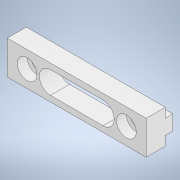
# Autodesk Inventor part: cameraModuleEnclosure
Saved by Autodesk Inventor 2022 (Build 260153000, 153)
## iProperties
Created: 2021-06-11
Part Number: cameraModuleEnclosure
Material: ABS Plastic
Document SubType Name: Modeling
Designer: tecware
Density: 1.06 g/cm^3
Appearance: Smooth - White
Mass: 91.0798 g
Surface Area: 506.315 cm^2
Volume: 85.9244 cm^3
Author: tecware
## iProperties of the stored document cameraModuleEnclosure_3DPrint.ipt
Created: 2021-06-17
Part Number: cameraModuleEnclosure_3DPrint
Material: Generic
Document SubType Name: Modeling
Designer: tecware
Density: 1 g/cm^3
Appearance: Default
Author: tecware
Autodesk Inventor part; units mm, degrees
ref_plane "YZ Plane" through (0, 0, 0) normal (1, 0, 0) x (0, 1, 0)
ref_plane "XZ Plane" through (0, 0, 0) normal (0, 1, 0) x (-1, 0, 0)
ref_plane "Work Plane15" through (0, 0, 83) normal (0, 0, 1) x (1, 0, 0)
sketch "Sketch35" plane through (0, 0, 83) normal (0, 0, 1) x (1, 0, 0)
  line L0 (-53.15, -19.2) -> (-22.85, -19.2)
  line L1 (-22.85, -19.2) -> (-22.85, -26.8)
  line L2 (-22.85, -26.8) -> (-53.15, -26.8)
  line L3 (-53.15, -26.8) -> (-53.15, -19.2)
  line L4 (-53.15, -26.8) -> (-22.85, -19.2) construction
  line L5 (-22.85, -26.8) -> (-53.15, -19.2) construction
  line L6 (-53.15, -23) -> (-49.35, -23) construction
  arc A0 (-49.35, -19.2) -> (-53.15, -23) centre (-49.35, -23) ccw
  arc A1 (-53.15, -23) -> (-49.35, -26.8) centre (-49.35, -23) ccw
  line L7 (-22.85, -23) -> (-26.65, -23) construction
  arc A2 (-22.85, -23) -> (-26.65, -19.2) centre (-26.65, -23) ccw
  arc A3 (-26.65, -26.8) -> (-22.85, -23) centre (-26.65, -23) ccw
  line L8 (-38, -26.8) -> (-38, -23)
  line L9 (-38, -26.8) -> (-34.2, -26.8) construction
  line L10 (-28, 6.8) -> (28, 6.8)
  line L11 (28, 6.8) -> (28, -6.8)
  line L12 (28, -6.8) -> (-28, -6.8)
  line L13 (-28, -6.8) -> (-28, 6.8)
  line L14 (-11.3, -22) -> (-6.85, -22) construction
  line L15 (3, -17.55) -> (3, -26.45)
  line L16 (-11.5, -17.5) -> (17.5, -17.5)
  line L17 (17.5, -17.5) -> (17.5, -26.5)
  line L18 (17.5, -26.5) -> (-11.5, -26.5)
  line L19 (-11.5, -26.5) -> (-11.5, -17.5)
  line L20 (-11.5, -22) -> (-7, -22)
  arc A4 (-7, -17.5) -> (-7, -26.5) centre (-7, -22) ccw
  arc A5 (13, -26.5) -> (13, -17.5) centre (13, -22) ccw
  line L21 (-15.1, 4.5) -> (15.1, 4.5)
  line L22 (15.1, 4.5) -> (15.1, -4.5)
  line L23 (15.1, -4.5) -> (-15.1, -4.5)
  line L24 (-15.1, -4.5) -> (-15.1, 4.5)
  line L25 (-15.1, 0) -> (-10.6, 0)
  arc A6 (-10.6, 4.5) -> (-10.6, -4.5) centre (-10.6, 0) ccw
  arc A7 (10.6, -4.5) -> (10.6, 4.5) centre (10.6, 0) ccw
  line L26 (0, 4.5) -> (0, -4.5)
  point P0 (0, 0)
  point P1 (69, 73)
  point P2 (-22.85, -23)
  point P3 (-22.85, -23)
  point P4 (-26.65, -26.8)
  point P5 (-26.65, -19.2)
  point P6 (13, -26.5)
  point P7 (13, -17.5)
  point P8 (0, 0)
  dimension "d253" = 7.6
  dimension "d265" = 3.8
  dimension "d316" = 3.8
  dimension "d317" = 90
  dimension "d359" = 29
  dimension "d360" = 9
  dimension "d361" = 4.5
  dimension "d362" = 30.2
  dimension "d363" = 9
  dimension "d364" = 4.5
  dimension "d365" = 56
  dimension "d366" = 13.6
  dimension "d367" = 2.3
  dimension "d368" = 12.9
  constraints: 54 end point, 18 point on circle, 9 horizontal, 8 centre point, 8 parallel, 8 point on line, 6 midpoint, 5 perpendicular, 3 symmetric about line, 2 coincident, 1 concentric, 1 other
  measures "d253" distance of L0.end L1.end
  measures "d265" distance of L6.start L6.end
  measures "d316" distance of L8.start L8.end
  measures "d317" angle of L9 L8
  measures "d359" distance of L17.end L18.end
  measures "d360" distance of L16.end L17.end
  measures "d361" distance of L20.start L20.end
  measures "d362" distance of L22.end L23.end
  measures "d363" distance of L21.end L22.end
  measures "d364" distance of L25.start L25.end
  measures "d365" distance of L10.start L10.end
  measures "d366" distance of L10.end L11.end
  measures "d367" distance between parallel lines of L21 L10
  measures "d368" distance between parallel lines of L11 L22
extrude "Extrusion25" add sketch "Sketch35" against normal blind 7.7 contours L10 L11 L12 L13 | L21 A6 L24 | A6 L23 L24 | L21 L22 A7 | L22 L23 A7
sketch "Sketch46" plane through (0, 0, 83) normal (0, 0, 1) x (1, 0, 0)
  point P0 (0, 0)
  point P1 (-20, 0)
  point P2 (20, 0)
hole "Hole8" at (20, 0, 83) at (-20, 0, 83) direction (0, 0, -1) diameter 4.2 depth 7.7 counterbore diameter 8 counterbore depth 4
sketch "Sketch47" plane through (0, 0, 75.3) normal (0, 0, -1) x (-1, 0, 0)
  line L0 (28, -3) -> (25, -3)
  line L1 (25, -3) -> (25, 3)
  line L2 (25, 3) -> (28, 3)
  line L3 (28, 3) -> (28, -3)
  line L4 (0, 0) -> (0, 11)
  line L5 (-28, -3) -> (-25, -3)
  line L6 (-25, -3) -> (-25, 3)
  line L7 (-25, 3) -> (-28, 3)
  line L8 (-28, 3) -> (-28, -3)
  line L9 (28, -6.8) -> (28, 6.8) projected
  dimension "d378" = 3
  dimension "d379" = 6
  dimension "d380" = 0
  constraints: 18 end point, 4 symmetric about line, 2 parallel, 1 horizontal, 1 perpendicular
  measures "d378" distance of L0.start L0.end
  measures "d379" distance of L0.end L1.end
  measures "d380" distance between parallel lines of L9 L3
extrude "Extrusion34" add sketch "Sketch47" along normal blind 3
body "Solid1"
